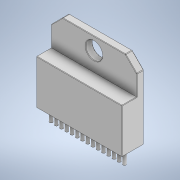
# Autodesk Inventor part: l298n
Saved by Autodesk Inventor 2020 (Build 240168000, 168)
## iProperties
Created: 2020-02-24
Part Number: l298n
Material: Типовые
Document SubType Name: Modeling
Designer: andrey
Density: 1 g/cm^3
Appearance: По умолчанию
Author: andrey
Autodesk Inventor part; units mm, degrees
ref_plane "YZ Plane" through (0, 0, 0) normal (1, 0, 0) x (0, 1, 0)
ref_plane "XZ Plane" through (0, 0, 0) normal (0, 1, 0) x (-1, 0, 0)
ref_plane "XY Plane" through (0, 0, 0) normal (0, 0, 1) x (1, 0, 0)
sketch "Эскиз1" plane through (0, 0, 0) normal (0, 0, 1) x (1, 0, 0)
  line L0 (0, 0) -> (19.6, 0)
  line L1 (19.6, 0) -> (19.6, 17.5)
  line L2 (19.6, 17.5) -> (0, 17.5)
  line L3 (0, 17.5) -> (0, 0)
  line L4 (0, 0) -> (0, 10.7)
  line L5 (0, 10.7) -> (19.6, 10.7)
  line L6 (19.6, 17.5) -> (17, 17.5)
  line L7 (19.6, 17.5) -> (19.6, 14.9)
  line L8 (19.6, 14.9) -> (17, 17.5)
  line L9 (0, 17.5) -> (2.6, 17.5)
  line L10 (0, 17.5) -> (0, 14.9)
  line L11 (0, 14.9) -> (2.6, 17.5)
  dimension "d0" = 19.6
  dimension "d1" = 17.5
  dimension "d2" = 10.7
  dimension "d3" = 2.6
  dimension "d4" = 2.6
  dimension "d5" = 2.6
  dimension "d6" = 2.6
  constraints: 24 end point, 6 point on line, 2 parallel, 2 perpendicular, 1 horizontal
  measures "d0" distance of L2.end L1.end
  measures "d1" distance of L1.end L0.end
  measures "d2" distance of L0.start L4.end
  measures "d3" distance of L1.end L6.end
  measures "d4" distance of L1.end L7.end
  measures "d5" distance of L2.end L9.end
  measures "d6" distance of L2.end L10.end
extrude "Выдавливание1" add sketch "Эскиз1" along normal blind 1.6 contours L3 L5 L1 L0 | L3 L11 L2 L8 L1 L5
sketch "Эскиз2" plane through (0, 0, 1.6) normal (0, 0, 1) x (1, 0, 0)
  line L0 (2.6, 17.5) -> (0, 14.9) projected
  line L1 (19.6, 0) -> (19.6, 14.9) projected
  line L2 (0, 14.9) -> (19.6, 14.9)
  line L3 (19.6, 14.9) -> (9.8, 14.9)
  line L4 (17, 17.5) -> (2.6, 17.5) projected
  line L5 (9.8, 17.5) -> (9.8, 14.6)
  circle A0 centre (9.8, 14.6) radius 1.925
  point P0 (0, 0)
  dimension "d9" = 2.9
  dimension "d10" = 3.85
  constraints: 6 end point, 2 midpoint, 1 centre point, 1 coincident, 1 horizontal, 1 vertical
  measures "d9" distance of L5.start L5.end
  measures "d10" diameter of A0
extrude "Выдавливание2" cut sketch "Эскиз2" against normal blind 1.6 contours A0 L5 L2 | L2 A0 | A0 L2 L5
sketch "Эскиз3" plane through (0, 0, 1.6) normal (0, 0, 1) x (1, 0, 0)
  line L0 (0, 14.9) -> (0, 0) projected
  line L1 (0, 0) -> (0, 10.3)
  line L2 (0, 0) -> (19.6, 0) projected
  line L3 (19.6, 0) -> (19.6, 10.3)
  line L4 (19.6, 0) -> (19.6, 14.9) projected
  line L5 (19.6, 10.3) -> (0, 10.3)
  dimension "d13" = 10.3
  dimension "d14" = 10.3
  constraints: 6 end point, 2 point on line
  measures "d13" distance of L0.end L1.end
  measures "d14" distance of L2.end L3.end
extrude "Выдавливание3" add sketch "Эскиз3" along normal blind 3.4
chamfer "Фаска1" distance 0.1 angle 45 1 edges at (9.8, 10.3, 5)
chamfer "Фаска2" distance 0.1 angle 45 16 edges at (19.6, 5.1, 5) (0, 5.1, 5) (9.8, 17.5, 1.6) (18.3, 16.2, 1.6) (19.6, 12.6, 1.6) (0, 12.6, 1.6) (1.3, 16.2, 1.6) (19.6, 14.9, 0.8) (17, 17.5, 0.8) (7.875, 14.6, 1.6) (7.875, 14.6, 0) (9.8, 17.5, 0) (18.3, 16.2, 0) (19.6, 7.45, 0) (19.6, 10.3, 3.25) (0, 10.3, 3.25)
chamfer "Фаска3" distance 0.2 angle 45 1 edges at (9.75, 0, 0)
chamfer "Фаска4" distance 0.2 angle 45 3 edges at (19.6, 0, 2.55) (0, 0, 2.55) (9.8, 0, 5)
chamfer "Фаска5" distance 0.1 angle 45 4 edges at (0, 7.55, 0) (1.25, 16.15, 0) (2.6, 17.5, 0.8) (0, 14.9, 0.75)
sketch "Эскиз4" plane through (0.2, 0, 4.8) normal (0, -1, 0) x (1, 0, 0)
  line L0 (0, -4.6) -> (0, 0) projected
  line L1 (19.2, 0) -> (19.2, -4.6) projected
  line L2 (0, 0) -> (19.2, 0)
  line L3 (19.2, 0) -> (19.2, -3.6)
  line L4 (19.2, -3.6) -> (0, -3.6)
  line L5 (0, -3.6) -> (0, 0)
  line L6 (-0.15, 0.15) -> (0, 0) projected
  line L7 (9.6, -1.8) -> (0, -1.8)
  line L8 (9.6, -1.8) -> (19.2, -1.8)
  line L9 (0, 0) -> (19.2, 0) projected
  line L10 (0, -3.6) -> (19.2, 0)
  line L11 (0, 0) -> (19.2, -3.6)
  line L12 (9.6, -1.8) -> (9.6, 0)
  line L13 (9.6, 0) -> (0, -3.6)
  line L14 (0, 0) -> (9.6, -3.6)
  line L15 (9.6, -3.6) -> (19.2, 0)
  line L16 (9.6, 0) -> (19.2, -3.6)
  line L17 (4.8, -1.8) -> (4.8, 0)
  line L18 (4.8, 0) -> (0, -3.6)
  line L19 (0, 0) -> (4.8, -3.6)
  line L20 (4.8, -3.6) -> (9.6, 0)
  line L21 (4.8, 0) -> (9.6, -3.6)
  line L22 (14.4, -1.8) -> (14.4, 0)
  line L23 (14.4, 0) -> (9.6, -3.6)
  line L24 (9.6, 0) -> (14.4, -3.6)
  line L25 (14.4, -3.6) -> (19.2, 0)
  line L26 (14.4, 0) -> (19.2, -3.6)
  line L27 (16.8, -1.8) -> (16.8, 0)
  line L28 (19.2, 0) -> (16.8, -3.6)
  line L29 (16.8, 0) -> (19.2, -3.6)
  line L30 (16.8, 0) -> (14.4, -3.6)
  line L31 (14.4, 0) -> (16.8, -3.6)
  line L32 (12, -1.8) -> (12, 0)
  line L33 (14.4, 0) -> (12, -3.6)
  line L34 (12, 0) -> (14.4, -3.6)
  line L35 (12, 0) -> (9.6, -3.6)
  line L36 (9.6, 0) -> (12, -3.6)
  line L37 (9.6, 0) -> (7.2, -3.6)
  line L38 (7.2, 0) -> (9.6, -3.6)
  line L39 (7.2, 0) -> (4.8, -3.6)
  line L40 (4.8, 0) -> (7.2, -3.6)
  line L41 (2.4, -1.8) -> (2.4, 0)
  line L42 (4.8, 0) -> (2.4, -3.6)
  line L43 (2.4, 0) -> (4.8, -3.6)
  line L44 (2.4, 0) -> (0, -3.6)
  line L45 (0, 0) -> (2.4, -3.6)
  circle A0 centre (1.2, -1.8) radius 0.35
  circle A1 centre (2.4, -1.8) radius 0.35
  circle A2 centre (3.6, -1.8) radius 0.35
  circle A3 centre (4.8, -1.8) radius 0.35
  circle A4 centre (6, -1.8) radius 0.35
  circle A5 centre (7.2, -1.8) radius 0.35
  circle A6 centre (8.4, -1.8) radius 0.35
  circle A7 centre (9.6, -1.8) radius 0.35
  circle A8 centre (10.8, -1.8) radius 0.35
  circle A9 centre (12, -1.8) radius 0.35
  circle A10 centre (13.2, -1.8) radius 0.35
  circle A11 centre (14.4, -1.8) radius 0.35
  circle A12 centre (15.6, -1.8) radius 0.35
  circle A13 centre (16.8, -1.8) radius 0.35
  circle A14 centre (18, -1.8) radius 0.35
  point P0 (-0.2, -4.8)
  dimension "d32" = 3.6
  dimension "d33" = 0.7
  dimension "d34" = 0.7
  dimension "d35" = 0.7
  dimension "d36" = 0.7
  dimension "d37" = 0.7
  dimension "d38" = 0.7
  dimension "d39" = 0.7
  dimension "d40" = 0.7
  dimension "d41" = 0.7
  dimension "d42" = 0.7
  dimension "d43" = 0.7
  dimension "d44" = 0.7
  dimension "d45" = 0.7
  dimension "d46" = 0.7
  dimension "d47" = 0.7
  constraints: 82 end point, 16 midpoint, 15 centre point, 13 parallel, 9 point on line, 6 coincident, 2 horizontal, 2 vertical, 1 perpendicular, 18 other
  measures "d32" distance of L2.end L3.end
  measures "d33" diameter of A0
  measures "d34" diameter of A1
  measures "d35" diameter of A2
  measures "d36" diameter of A3
  measures "d37" diameter of A4
  measures "d38" diameter of A5
  measures "d39" diameter of A6
  measures "d40" diameter of A7
  measures "d41" diameter of A8
  measures "d42" diameter of A9
  measures "d43" diameter of A10
  measures "d44" diameter of A11
  measures "d45" diameter of A12
  measures "d46" diameter of A13
  measures "d47" diameter of A14
extrude "Выдавливание4" add sketch "Эскиз4" along normal blind 3 contours A0 L7 L44 | L44 L45 A0 | A0 L45 L7 | A1 L7 L18 | L18 L19 A1 | L45 L7 A0 | L44 A0 L7 | L45 A0 L44 | L19 L7 A1 | A2 L7 L42 | L42 L43 A2 | L18 A1 L7 | L41 A1 L18 | L7 A1 L19 | L19 A1 L41 | A5 L7 L20 | L20 L21 A5 | A4 L39 L40 | L40 L7 A4 | A3 L7 L13 | L13 L14 A3 | L43 L7 A2 | L42 A2 L7 | L43 A2 L42 | L7 A2 L43 | A8 L11 L35 | L35 L11 L36 A8 | A6 L37 L10 L38 | L38 L10 A6 | A6 L7 L37 L10 | L10 L37 A6 | L21 L7 A5 | L14 L7 A3 | A4 L7 L39 | L20 A5 L7 | L21 A5 L20 | L7 A5 L21 | L39 A4 L7 | L40 A4 L39 | L7 A4 L40 | L13 A3 L7 | L17 A3 L13 | L7 A3 L14 | L14 A3 L17 | L36 L11 A8 | L35 L36 L11 | L11 A8 L8 L35 | L38 L7 A6 L10 | L10 L37 L38 | A6 L11 L38 L7 | A7 L10 L12 | L12 L11 A7 | A8 L35 L10 L36 | L36 L10 A8 | A6 L11 L37 | L37 L11 L38 A6 | A6 L38 L11 | A9 L23 L24 | L24 L8 A9 | A10 L8 L33 | L33 L34 A10 | L11 L36 L8 A8 | A9 L8 L23 | L35 L10 A8 L8 | L36 L10 L35 | L8 A8 L10 L36 | A7 L10 L11 | L11 L8 A7 | L37 L11 A6 L7 | L38 L11 L37 | A7 L7 L10 | L10 A7 L8 | L7 A7 L11 | A8 L10 L35 | A11 L8 L15 | L15 L16 A11 | L34 L8 A10 | L23 A9 L8 | L32 A9 L23 | L8 A9 L24 | L24 A9 L32 | L33 A10 L8 | L34 A10 L33 | L8 A10 L34 | A14 L28 L29 | L29 L8 A14 | A13 L8 L25 | L25 L26 A13 | A12 L30 L31 | L31 L8 A12 | L16 L8 A11 | A12 L8 L30 | L15 A11 L8 | L22 A11 L15 | L8 A11 L16 | L16 A11 L22 | L8 L28 A14 | L26 L8 A13 | A14 L8 L28 | L29 A14 L28 | L8 A14 L29 | L25 A13 L8 | L27 A13 L25 | L8 A13 L26 | L26 A13 L27 | L30 A12 L8 | L31 A12 L30 | L8 A12 L31
sketch "Эскиз5" plane through (1.4, -3, 3) normal (0, -1, 0) x (1, 0, 0)
  point P0 (-1.4, -3)
